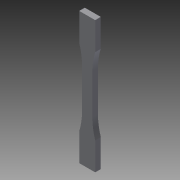
# Autodesk Inventor part: Generic DogBone
Saved by Autodesk Inventor 2014 SP1 (Build 180222100, 222)
## iProperties
Created: 2015-01-22
Part Number: Generic DogBone
Material: Generic
Document SubType Name: Modeling
Designer: Nick
Density: 1 g/cm^3
Appearance: Default
Author: Nick
Autodesk Inventor part; units mm, degrees
ref_plane "YZ Plane" through (0, 0, 0) normal (1, 0, 0) x (0, 1, 0)
ref_plane "XZ Plane" through (0, 0, 0) normal (0, 1, 0) x (-1, 0, 0)
ref_plane "XY Plane" through (0, 0, 0) normal (0, 0, 1) x (1, 0, 0)
sketch "Sketch1" plane through (0, 0, 0) normal (0, 1, 0) x (-1, 0, 0)
  line L0 (0, 0) -> (20, 0)
  line L1 (3.5, 57.5) -> (3.5, 82.5)
  line L2 (16.5, 57.5) -> (16.5, 82.5)
  arc A0 (16.5, 57.5) -> (20, 34.702) centre (92.5, 57.5) ccw
  arc A1 (0, 34.702) -> (3.5, 57.5) centre (-72.5, 57.5) ccw
  line L3 (3.5, 82.5) -> (16.5, 82.5) construction
  line L4 (0, 34.702) -> (0, 0)
  line L5 (20, 34.702) -> (20, 0)
  line L6 (0, 165) -> (20, 165)
  line L7 (3.5, 107.5) -> (3.5, 82.5)
  line L8 (16.5, 107.5) -> (16.5, 82.5)
  arc A2 (20, 130.298) -> (16.5, 107.5) centre (92.5, 107.5) ccw
  arc A3 (3.5, 107.5) -> (0, 130.298) centre (-72.5, 107.5) ccw
  line L9 (0, 130.298) -> (0, 165)
  line L10 (20, 130.298) -> (20, 165)
  dimension "d2" = 20
  dimension "d5" = 76
  dimension "d6" = 76
  dimension "d7" = 82.5
  dimension "d8" = 13
  dimension "d9" = 25
  constraints: 22 end point, 8 point on circle, 8 symmetric about line, 4 centre point, 2 parallel, 2 perpendicular, 2 tangent, 2 vertical alignment, 1 horizontal alignment, 1 vertical, 2 other
  measures "d2" distance of L0.start L0.end
  measures "d5" radius of A0
  measures "d6" radius of A1
  measures "d7" distance between parallel lines of L0 L3
  measures "d8" distance between parallel lines of L2 L1
  measures "d9" distance of L1.start L1.end
extrude "Extrusion1" add sketch "Sketch1" along normal blind 7
body "Solid1"
